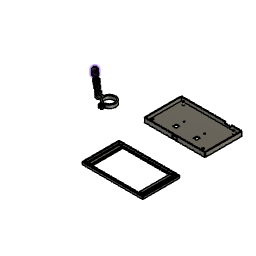
Mount_Nextion_Display v32 (Autodesk Fusion 360 design; units mm, degrees)
Autodesk Fusion 360 part; units mm, degrees
note: some values were not read from the file. Chosen so that the rebuilt part matches the saved one: which face or edge a step refers to. Set by a fixed rule: which sketch regions a step uses.
sketch "Skizze1" plane through (0, 0, 0) normal (0, 0, 1) x (1, 0, 0)
  line L0 (-15.9925, -2.25) -> (-31.6304, -2.25)
  line L1 (-29.9925, 2.25) -> (-15.9925, 2.25)
  line L2 (-31.6304, -2.25) -> (-86.5082, 43.7979)
  line L3 (-86.5082, 43.7979) -> (-83.6156, 47.2451)
  line L4 (-1, -23.6468) -> (-4, -23.6468)
  line L5 (-4, -23.6468) -> (-4, -15.6468)
  line L6 (-1, -23.6468) -> (-1, -12.6104)
  arc A0 (-15.9925, -2.25) -> (-4, -15.6468) centre (0, 0) ccw
  arc A1 (4, -15.6468) -> (-15.9925, 2.25) centre (0, 0) ccw
  line L7 (1, -12.6104) -> (1, -23.6468)
  line L8 (4, -15.6468) -> (4, -23.6468)
  line L9 (4, -23.6468) -> (1, -23.6468)
  arc A2 (1, -12.6104) -> (-1, -12.6104) centre (0, 0) ccw
  line L10 (-29.9925, 2.25) -> (-50.4157, 19.3871)
  line L11 (-57.0334, 24.94) -> (-83.6156, 47.2451)
  line L12 (-57.0334, 24.94) -> (-50.4157, 19.3871)
  dimension "d3" = 25.3
  dimension "d7" = 4.5
  dimension "d8" = 2.25
  dimension "d10" = 140
  dimension "d11" = 90
  dimension "d12" = 4.5
  dimension "d13" = 70
  dimension "d14" = 14
  dimension "d19" = 8
  dimension "d22" = 1
  dimension "d23" = 3
  dimension "d24" = 8
  dimension "d26" = 3
  dimension "d27" = 1
  dimension "d48" = 3.5
  dimension "d49" = 3.5
  constraint coincident A0.centre A1.centre
  constraint concentric A0 A2
  constraint horizontal L0
  constraint parallel L2 L10
  constraint perpendicular L4 L5
  constraint perpendicular L4 L6
  constraint concentric A0 A1
  constraint vertical L7
  constraint vertical L6
  constraint vertical L8
  constraint perpendicular L7 L9
  constraint coincident L11.start L10
  constraint collinear L10 L11
  measures "d3" diameter of A2
  measures "d7" distance of L0 L1
  measures "d8" distance of A0.centre L1
  measures "d10" angle of L1 L10
  measures "d11" angle of L3 L10
  measures "d12" distance of L2 L10
  measures "d13" distance of L1.start L3.end
  measures "d14" distance of L1.start L1.end
  measures "d19" distance of L4.end L5.end
  measures "d22" distance of A0.centre L6
  measures "d23" distance of L4.start L4.end
  measures "d24" distance of A1.start L8.end
  measures "d26" distance of L7.end L8.end
  measures "d27" distance of A0.centre L7
  measures "d48" distance of A0 A2
  measures "d49" distance of A1 A2
extrude "Extrusion1" add sketch "Skizze1" along normal blind 8 makes body 1
sketch "Skizze2" plane through (4, 0, 0) normal (1, 0, 0) x (0, 1, 0)
  line L0 (-23.6468, 0) -> (-15.6468, 0)
  line L1 (-15.6468, 0) -> (-15.6468, 8)
  line L2 (-15.6468, 8) -> (-23.6468, 8)
  line L3 (-23.6468, 8) -> (-23.6468, 0)
  line L4 (-23.6468, 8) -> (-15.6468, 0) construction
  line L5 (-15.6468, 8) -> (-23.6468, 0) construction
  circle A0 centre (-19.6468, 4) radius 1.5
  dimension "d28" = 3
  constraint coincident L2.end L3.start
  constraint coincident L0.end L1.start
  constraint coincident L1.end L2.start
  constraint coincident L0.start L3.end
  constraint midpoint L4 A0.centre
  measures "d28" diameter of A0
extrude "Extrusion2" cut sketch "Skizze2" against normal up to surface (8 mm away) contours A0 bodies 1
sketch "Skizze3" plane through (-11.2843, -13.4481, 0) normal (0.642788, 0.766044, 0) x (-0.766044, 0.642788, 0)
  line L0 (24.4219, 0) -> (94.4219, 0)
  line L1 (94.4219, 0) -> (94.4219, 8)
  line L2 (94.4219, 8) -> (24.4219, 8)
  line L3 (24.4219, 8) -> (24.4219, 0)
  circle A0 centre (46.9219, 4) radius 1.75
  line L4 (24.4219, 8) -> (94.4219, 0) construction
  line L5 (94.4219, 8) -> (24.4219, 0) construction
  line L6 (59.4219, 4) -> (24.4219, 4) construction
  line L7 (59.4219, 4) -> (94.4219, 4) construction
  circle A1 centre (86.9219, 4) radius 1.75
  line L8 (62.4219, 8) -> (71.4219, 8)
  line L9 (71.4219, 8) -> (71.4219, 0)
  line L10 (71.4219, 0) -> (62.4219, 0)
  line L11 (62.4219, 0) -> (62.4219, 8)
  line L12 (62.4219, 8) -> (71.4219, 0) construction
  line L13 (71.4219, 8) -> (62.4219, 0) construction
  point P0 (59.4219, 4)
  point P1 (66.9219, 4)
  dimension "d34" = 3.5
  dimension "d35" = 3.5
  dimension "d50" = 22.5
  dimension "d68" = 40
  dimension "d164" = 20
  dimension "d165" = 9
  constraint coincident L2.end L3.start
  constraint coincident L0.end L1.start
  constraint coincident L1.end L2.start
  constraint coincident L0.start L3.end
  constraint midpoint L4 P0
  constraint horizontal L6
  constraint midpoint L3 L6.end
  constraint midpoint L1 L7.end
  constraint coincident A0.centre L6
  constraint coincident L7 A1.centre
  constraint coincident P0 L6.start
  constraint horizontal L8
  constraint perpendicular L8 L9
  constraint parallel L8 L10
  constraint parallel L9 L11
  constraint coincident L2 L8.start
  constraint coincident L12 P1
  constraint coincident L13 P1
  constraint coincident L7 P1
  measures "d34" diameter of A0
  measures "d35" diameter of A1
  measures "d50" distance of L3 A0.centre
  measures "d68" distance of A0.centre A1.centre
  measures "d164" distance of A0.centre P1
  measures "d165" distance of L9 L11
extrude "Extrusion3" cut sketch "Skizze3" against normal up to surface (4.5 mm away) contours A0 | A1 bodies 1
extrude "Extrusion10" add sketch "Skizze3" along normal blind 2 contours L0 L2 L8 L9 L10 L11 bodies 1
sketch "Skizze14" plane through (0, 0, 8) normal (0, 0, 1) x (-1, 0, 0)
  line L0 (31.6304, 2.25) -> (15.9925, 2.25)
  arc A0 (15.9925, 2.25) -> (4, 15.6468) centre (0, 0) ccw
  line L1 (4, 15.6468) -> (4, 23.6468)
  line L2 (4, 23.6468) -> (1, 23.6468)
  line L3 (1, 23.6468) -> (1, 12.6104)
  arc A1 (-1, 12.6104) -> (1, 12.6104) centre (0, 0) ccw
  line L4 (-1, 12.6104) -> (-1, 23.6468)
  line L5 (-1, 23.6468) -> (-4, 23.6468)
  line L6 (-4, 23.6468) -> (-4, 15.6468)
  line L7 (15.9925, -2.25) -> (29.9925, -2.25)
  line L8 (29.9925, -2.25) -> (59.1022, -26.6759)
  line L9 (59.1022, -26.6759) -> (57.8166, -28.208)
  line L10 (57.8166, -28.208) -> (64.711, -33.9931)
  line L11 (64.711, -33.9931) -> (65.9966, -32.461)
  line L12 (65.9966, -32.461) -> (83.6156, -47.2451)
  line L13 (83.6156, -47.2451) -> (86.5082, -43.7979)
  line L14 (86.5082, -43.7979) -> (31.6304, 2.25)
  line L15 (29.9925, -2.25) -> (32.885, 1.1972) construction
  line L16 (29.9925, -2.25) -> (83.6156, -47.2451)
  line L17 (43.7813, -13.8202) -> (46.6738, -10.373)
  arc A2 (-4, 15.6468) -> (15.9925, -2.25) centre (0, 0) ccw
  dimension "d174" = 18
  constraint coincident L7.end L8.start
  constraint coincident L14 L15.end
  constraint perpendicular L15 L16
  constraint coincident L16 L17.start
  constraint coincident L14 L17.end
  constraint perpendicular L14 L17
  measures "d174" distance of L15 L17
extrude "Extrusion11" add sketch "Skizze14" along normal blind 2 contours L8 L12 L13 L14 L16 L17 bodies 1
fillet "Abrundung2" radius 1 4 edges at (-15.9925, -2.25, 4) (-15.9925, 2.25, 4) (-4, -15.6468, 4) (4, -15.6468, 4) on bodies 1
fillet "Abrundung2" radius 2 2 edges at (-31.6304, -2.25, 4) (-29.9925, 2.25, 4) on bodies 1
sketch "Skizze5" plane through (0, 0, 0) normal (0, 0, 1) x (1, 0, 0)
  circle A0 centre (135.6, 52.4) radius 1.75
  circle A1 centre (135.6, 12.4) radius 1.75
  line L0 (161.6, 91.4) -> (161.6, 7.4) construction
  circle A2 centre (187.6, 12.4) radius 1.75
  circle A3 centre (187.6, 52.4) radius 1.75
  line L1 (228.35, 7.4) -> (94.85, 7.4) construction
  line L2 (94.85, 7.4) -> (94.85, 91.4) construction
  line L3 (94.85, 91.4) -> (228.35, 91.4) construction
  line L4 (228.35, 91.4) -> (228.35, 7.4) construction
  line L5 (228.35, 7.4) -> (94.85, 91.4) construction
  line L6 (94.85, 7.4) -> (228.35, 91.4) construction
  circle A4 centre (225.15, 88.2) radius 1.6
  circle A5 centre (225.15, 88.2) radius 2.6
  line L7 (161.6, 49.4) -> (228.35, 49.4) construction
  circle A6 centre (225.15, 10.6) radius 2.6
  circle A7 centre (225.15, 10.6) radius 1.6
  circle A8 centre (98.05, 88.2) radius 2.6
  circle A9 centre (98.05, 88.2) radius 1.6
  circle A10 centre (98.05, 10.6) radius 2.6
  circle A11 centre (98.05, 10.6) radius 1.6
  line L8 (86.85, 94.4) -> (236.35, 94.4)
  line L9 (236.35, 94.4) -> (236.35, 4.4)
  line L10 (236.35, 4.4) -> (86.85, 4.4)
  line L11 (86.85, 4.4) -> (86.85, 94.4)
  line L12 (238.35, 2.4) -> (84.85, 2.4)
  line L13 (84.85, 2.4) -> (84.85, 96.4)
  line L14 (84.85, 96.4) -> (238.35, 96.4)
  line L15 (238.35, 96.4) -> (238.35, 2.4)
  line L16 (135.6, 52.4) -> (135.6, 12.4) construction
  line L17 (131.5, 37) -> (139.7, 37)
  line L18 (139.7, 37) -> (139.7, 27.8)
  line L19 (139.7, 27.8) -> (131.5, 27.8)
  line L20 (131.5, 27.8) -> (131.5, 37)
  line L21 (131.5, 37) -> (139.7, 27.8) construction
  line L22 (139.7, 37) -> (131.5, 27.8) construction
  line L23 (183.5, 27.8) -> (191.7, 27.8)
  line L24 (191.7, 27.8) -> (191.7, 37)
  line L25 (191.7, 37) -> (183.5, 37)
  line L26 (183.5, 37) -> (183.5, 27.8)
  point P0 (161.6, 49.4)
  point P1 (135.6, 32.4)
  point P2 (135.6, 32.4)
  dimension "d54" = 3.5
  dimension "d55" = 3.5
  dimension "d56" = 40
  dimension "d71" = 26
  dimension "d73" = 26
  dimension "d74" = 133.5
  dimension "d75" = 84
  dimension "d76" = 5
  dimension "d77" = 38.8
  dimension "d78" = 3.2
  dimension "d79" = 63.55
  dimension "d80" = 1
  dimension "d91" = 8
  dimension "d92" = 8
  dimension "d93" = 3
  dimension "d94" = 3
  dimension "d95" = -2
  dimension "d168" = 8.2
  dimension "d169" = 9.2
  constraint symmetric A0 L0 A3
  constraint symmetric A1 L0 A2
  constraint horizontal L1
  constraint perpendicular L1 L2
  constraint parallel L1 L3
  constraint parallel L2 L4
  constraint coincident L5 P0
  constraint coincident L6 P0
  constraint midpoint L0 P0
  constraint midpoint L0.start L3
  constraint coincident P0 L7.start
  constraint perpendicular L4 L7
  constraint midpoint L4 L7.end
  constraint symmetric A4 L7 A7
  constraint symmetric A5 L7 A6
  constraint symmetric L0 A4 A9
  constraint symmetric L0 A5 A8
  constraint symmetric L0 A6 A10
  constraint symmetric L0 A7 A11
  constraint horizontal L8
  constraint vertical L9
  constraint horizontal L10
  constraint vertical L11
  constraint coincident A0.centre L16.start
  constraint coincident A1.centre L16.end
  constraint midpoint L16 P2
  constraint horizontal L17
  constraint perpendicular L17 L18
  constraint parallel L17 L19
  constraint parallel L18 L20
  constraint coincident L21 P2
  constraint coincident L22 P2
  constraint coincident P2 P1
  constraint symmetric L0 L17.start L24.end
  constraint symmetric L0 L17.end L25.end
  constraint symmetric L0 L18.end L23.start
  constraint symmetric L0 L19.end L23.end
  measures "d54" diameter of A1
  measures "d55" diameter of A0
  measures "d56" vertical distance of A0.centre A1.centre
  measures "d71" distance of A0.centre L0
  measures "d73" distance of A1.centre L0
  measures "d74" distance of L2.end L3.end
  measures "d75" distance of L1.end L2.end
  measures "d76" distance of A1.centre L1
  measures "d77" vertical distance of P0 A4.centre
  measures "d78" diameter of A4
  measures "d79" horizontal distance of P0 A4.centre
  measures "d91" distance of L4 L9
  measures "d92" distance of L2 L11
  measures "d93" distance of L1 L10
  measures "d94" distance of L3 L8
  measures "d168" distance of L18.end L19.end
  measures "d169" distance of L17.end L18.end
extrude "Extrusion4" add sketch "Skizze5" along normal blind 2 separate body contours L8 L9 L10 L11 makes body 2
extrude "Extrusion5" add sketch "Skizze5" along normal blind 9 contours A5 | A6 | A8 | A10 bodies 2
extrude "Extrusion6" add sketch "Skizze5" along normal blind 10.7 contours L12 L13 L14 L15 bodies 2
sketch "Skizze13" plane through (0, 4.4, 0) normal (0, 1, 0) x (-1, 0, 0)
  line L0 (-236.35, 2) -> (-86.85, 2)
  line L1 (-86.85, 2) -> (-86.85, 10.7)
  line L2 (-86.85, 10.7) -> (-236.35, 10.7)
  line L3 (-236.35, 10.7) -> (-236.35, 2)
  line L4 (-161.6, 2) -> (-161.6, 10.7) construction
  line L5 (-167.8, 8.2) -> (-155.4, 8.2)
  line L6 (-155.4, 8.2) -> (-155.4, 2)
  line L7 (-155.4, 2) -> (-167.8, 2)
  line L8 (-167.8, 2) -> (-167.8, 8.2)
  dimension "d159" = 12.4
  dimension "d160" = 6.2
  constraint midpoint L0 L4.start
  constraint midpoint L2 L4.end
  constraint horizontal L5
  constraint vertical L6
  constraint horizontal L7
  constraint vertical L8
  constraint coincident L0 L6.end
  constraint symmetric L4 L6 L8
  measures "d159" distance of L5.start L5.end
  measures "d160" distance of L5.start L7.end
sketch "Skizze15" plane through (0, 94.4, 0) normal (0, -1, 0) x (1, 0, 0)
  line L0 (86.85, 2) -> (236.35, 2)
  line L1 (236.35, 2) -> (236.35, 10.7)
  line L2 (236.35, 10.7) -> (86.85, 10.7)
  line L3 (86.85, 10.7) -> (86.85, 2)
  line L4 (161.6, 10.7) -> (161.6, 2) construction
  line L5 (195.85, 10.7) -> (211.85, 10.7)
  line L6 (211.85, 10.7) -> (211.85, 6.5)
  line L7 (211.85, 6.5) -> (195.85, 6.5)
  line L8 (195.85, 6.5) -> (195.85, 10.7)
  dimension "d181" = 50.25
  dimension "d182" = 16
  dimension "d183" = 4.2
  constraint midpoint L2 L4.start
  constraint midpoint L0 L4.end
  constraint horizontal L5
  constraint vertical L6
  constraint horizontal L7
  constraint vertical L8
  constraint collinear L2 L5
  measures "d181" distance of L4 L6
  measures "d182" distance of L5.start L5.end
  measures "d183" distance of L5 L7
extrude "Extrusion9" cut sketch "Skizze13" against normal up to surface (2 mm away) contours L0 L5 L6 L7 L8 bodies 2
extrude "Extrusion12" cut sketch "Skizze15" against normal up to surface (2 mm away) contours L2 L5 L6 L7 L8 bodies 2
sketch "Skizze11" plane through (0, 0, 0) normal (0, 0, 1) x (1, 0, 0)
  line L0 (241.2112, -78.3101) -> (241.2112, -162.3101) construction
  line L1 (97.7112, -167.3101) -> (97.7112, -73.3101)
  circle A0 centre (110.8272, -81.8132) radius 1.6
  line L2 (107.7112, -162.3101) -> (107.7112, -78.3101) construction
  line L3 (251.2112, -73.3101) -> (251.2112, -167.3101)
  circle A1 centre (111.1967, -159.4123) radius 1.6
  line L4 (174.5612, -120.3101) -> (241.2112, -120.3101) construction
  line L5 (249.2112, -75.3101) -> (249.2112, -165.3101) construction
  circle A2 centre (238.1112, -81.5101) radius 1.6
  line L6 (99.7112, -165.3101) -> (99.7112, -75.3101) construction
  line L7 (99.7112, -75.3101) -> (249.2112, -75.3101) construction
  line L8 (251.2112, -167.3101) -> (97.7112, -167.3101)
  line L9 (174.4612, -78.3101) -> (174.6612, -162.3101) construction
  line L10 (97.7112, -73.3101) -> (251.2112, -73.3101)
  line L11 (241.2112, -162.3101) -> (107.7112, -162.3101) construction
  circle A3 centre (238.1112, -159.1101) radius 1.6
  line L12 (107.7112, -78.3101) -> (241.2112, -78.3101) construction
  line L13 (249.2112, -165.3101) -> (99.7112, -165.3101) construction
  line L14 (234.4112, -159.4101) -> (114.7112, -81.2101) construction
  line L15 (114.7112, -159.4101) -> (234.4112, -81.2101) construction
  line L16 (99.9112, -165.1101) -> (99.9112, -75.5101)
  line L17 (99.9112, -75.5101) -> (249.0112, -75.5101)
  line L18 (249.0112, -75.5101) -> (249.0112, -165.1101)
  line L19 (249.0112, -165.1101) -> (99.9112, -165.1101)
  line L20 (101.7112, -163.3101) -> (101.7112, -77.3101)
  line L21 (101.7112, -77.3101) -> (247.2112, -77.3101)
  line L22 (247.2112, -77.3101) -> (247.2112, -163.3101)
  line L23 (247.2112, -163.3101) -> (101.7112, -163.3101)
  line L24 (235.2112, -81.5101) -> (235.2112, -159.1101)
  line L25 (241.011, -81.539) -> (241.0112, -159.1101)
  arc A4 (241.011, -81.539) -> (235.2112, -81.5101) centre (238.1112, -81.5101) ccw
  arc A5 (235.2112, -159.1101) -> (241.0112, -159.1101) centre (238.1112, -159.1101) ccw
  line L26 (107.9275, -81.8559) -> (108.2967, -159.4261)
  arc A6 (113.7271, -81.7994) -> (107.9275, -81.8559) centre (110.8272, -81.8132) ccw
  line L27 (113.7271, -81.7994) -> (114.0966, -159.3985)
  arc A7 (108.2967, -159.4261) -> (114.0966, -159.3985) centre (111.1967, -159.4123) ccw
  line L28 (114.7112, -80.7101) -> (234.4112, -80.7101)
  line L29 (234.4112, -80.7101) -> (234.4112, -159.1101)
  line L30 (234.4112, -159.1101) -> (114.7112, -159.1101)
  line L31 (114.7112, -159.1101) -> (114.7112, -80.7101)
  point P0 (174.5612, -120.3101)
  point P1 (174.5612, -120.3101)
  dimension "d114" = 1
  dimension "d115" = -2
  dimension "d121" = 133.5
  dimension "d122" = 84
  dimension "d124" = 38.8
  dimension "d125" = 3.2
  dimension "d126" = 63.55
  dimension "d127" = 8
  dimension "d128" = 8
  dimension "d129" = 3
  dimension "d130" = 3
  dimension "d131" = 119.7
  dimension "d132" = 78.2
  dimension "d133" = 0.2
  dimension "d134" = 2
  dimension "d191" = 59.85
  dimension "d192" = 119.7
  dimension "d193" = 119.7
  dimension "d194" = 59.85
  dimension "d195" = 39.6
  dimension "d196" = 38.8
  constraint horizontal L11
  constraint perpendicular L2 L11
  constraint parallel L11 L12
  constraint parallel L0 L2
  constraint midpoint P1 L9
  constraint midpoint L9.start L12
  constraint coincident P1 P0
  constraint perpendicular L0 L4
  constraint midpoint L4.end L0
  constraint symmetric L4 A2 A3
  constraint symmetric A0 A2 L9
  constraint symmetric A1 L9 A3
  constraint horizontal L7
  constraint vertical L5
  constraint horizontal L13
  constraint vertical L6
  constraint coincident L14 P1
  constraint coincident L15 P1
  constraint tangent L24 A5
  constraint tangent L25 A5
  constraint concentric A2 A4
  constraint concentric A3 A5
  constraint symmetric L9 L24.start A6.start
  constraint symmetric L9 L24.end L27.end
  constraint symmetric L9 L25.start L26.start
  constraint symmetric L9 L25.end L26.end
  constraint symmetric L9 A4 A6
  constraint symmetric L9 A5 A7
  constraint horizontal L28
  constraint vertical L29
  constraint horizontal L30
  constraint vertical L31
  measures "d121" distance of L2.end L0.start
  measures "d122" distance of L2.start L2.end
  measures "d124" vertical distance of A2.centre P1
  measures "d125" diameter of A2
  measures "d126" horizontal distance of A2.centre P1
  measures "d127" distance of L0 L5
  measures "d128" distance of L2 L6
  measures "d129" distance of L11 L13
  measures "d130" distance of L7 L12
  measures "d131" distance of L14.end L15.end
  measures "d132" distance of L15.start L14.end
  measures "d191" distance of P1 L29
  measures "d192" distance of L14.start L15.start
  measures "d193" distance of L14.end L15.end
  measures "d194" distance of P1 L31
  measures "d195" distance of P1 L28
  measures "d196" distance of P1 L30
extrude "Extrusion7" add sketch "Skizze11" along normal blind 5 separate body contours L1 L3 L8 L10 | L24 L25 A4 A5 | L26 A6 L27 A7 makes body 3 at (109.3846, -107.7387, 0) makes body 4 at (199.3112, -166.5768, 0) makes body 5 at (235.8453, -107.7938, 0)
extrude "Extrusion13" add sketch "Skizze11" along normal blind 2 contours L20 L21 L22 L23 bodies 3 5
extrude "Extrusion8" add sketch "Skizze11" along normal blind 6.5 contours L16 L17 L18 L19 bodies 3 4
fillet "Abrundung3" radius 1.5 4 edges at (97.7112, -167.3101, 2.5) (97.7112, -73.3101, 2.5) (251.2112, -73.3101, 2.5) (251.2112, -167.3101, 2.5) on bodies 2 3
fillet "Abrundung3" radius 1.5 4 edges at (238.35, 2.4, 5.35) (238.35, 96.4, 5.35) (84.85, 96.4, 5.35) (84.85, 2.4, 5.35) on bodies 2 3
fillet "Abrundung4" radius 3 2 edges at (-45.2276, 12.0966, 10) (-45.2276, 12.0966, 8) on bodies 1
equation "lenker_außen_außendurchmesser = 22.2 mm"
equation "lenker_mitte_außendurchmesser = 25.3 mm"
equation "d3 = lenker_mitte_außendurchmesser"
equation "d8 = d7 / 2"
equation "d15 = breite_Halter"
equation "d24 = d19"
equation "d25 = ( d3 + 5 mm ) / 2"
equation "d26 = d23"
equation "d27 = d22"
equation "d34 = Durchmesser_Verbinder_Loecher"
equation "d35 = d34"
equation "Abstand_Verbinder_Loecher = 40 mm"
equation "Durchmesser_Verbinder_Loecher = 3.5 mm"
equation "d54 = Durchmesser_Verbinder_Loecher"
equation "d55 = Durchmesser_Verbinder_Loecher"
equation "d56 = Abstand_Verbinder_Loecher"
equation "d68 = Abstand_Verbinder_Loecher"
equation "breite_Halter = 8 mm"
equation "Breite_Mitte_Lenker = 45 mm" comment "Breite des Lenker-Risers"
equation "d71 = 30 mm - 4 mm"
equation "d73 = d71"
equation "d77 = ( 77.6 / 2 ) * 1 mm"
equation "d78 = 2 * 1.6 mm"
equation "d79 = ( 127.1 / 2 ) * 1 mm"
equation "d85 = Tiefe_Backplane - 1.7 mm"
equation "d87 = Tiefe_Backplane"
equation "d92 = d91"
equation "Tiefe_Backplane = 1.7 mm + 7 mm + 2 mm"
equation "d124 = ( 77.6 / 2 ) * 1 mm"
equation "d125 = 2 * 1.6 mm"
equation "d126 = ( 127.1 / 2 ) * 1 mm"
equation "d128 = d127"
equation "d164 = d68 / 2"
equation "d181 = ( 133.5 / 2 ) * 1 mm - 16.5 mm"
equation "d191 = ( 119.7 / 2 ) * 1 mm"
equation "d194 = d131 / 2"
equation "d195 = ( 78.2 / 2 ) * 1 mm + 0.5 mm"
equation "d196 = ( 78.2 / 2 ) * 1 mm - 0.3 mm"
named bodies: "mount", "Top Cover", "Back plate"
